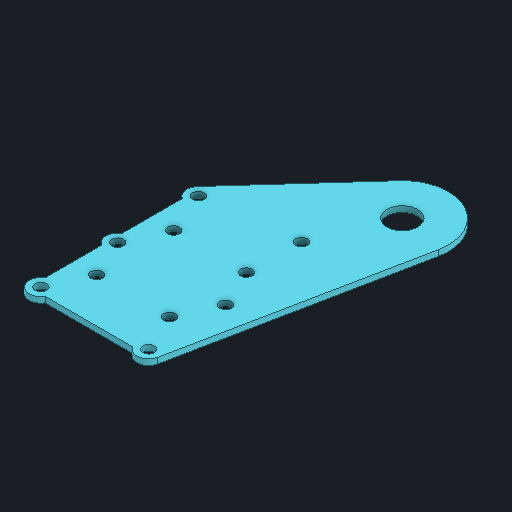
# Autodesk Inventor part: femur_support_steel
Saved by Autodesk Inventor 2026 (Build 300175000, 175)
## iProperties
Created: 2026-04-24
Part Number: femur_support_steel
Material: Сталь
Document SubType Name: Modeling
Designer: user
Density: 7.85 g/cm^3
Appearance: Серо-синий
Mass: 237.917 g
Surface Area: 222.677 cm^2
Volume: 30.3078 cm^3
Author: user
Autodesk Inventor part; units mm, degrees
ref_plane "YZ Plane" through (0, 0, 0) normal (1, 0, 0) x (0, 1, 0)
ref_plane "XZ Plane" through (0, 0, 0) normal (0, 1, 0) x (-1, 0, 0)
ref_plane "XY Plane" through (0, 0, 0) normal (0, 0, 1) x (1, 0, 0)
sketch "Эскиз1" plane through (0, 0, 0) normal (0, 1, 0) x (-1, 0, 0)
  circle A0 centre (41.8656, -145.8142) radius 8
  line L0 (111.6413, -105.8142) -> (38.7953, -105.8142) construction
  line L1 (76.8656, 21.9817) -> (76.8656, -112.0617)
  circle A1 centre (48.8156, -20.8142) radius 3.05
  circle A2 centre (57.9156, -40.8142) radius 3.05
  circle A3 centre (48.8156, -60.8142) radius 3.05
  circle A4 centre (57.9156, -80.8142) radius 3.05
  circle A5 centre (57.3656, -108.8642) radius 3.05
  circle A6 centre (104.9156, -102.7642) radius 3.05
  circle A7 centre (95.8156, -80.8142) radius 3.05
  circle A8 centre (104.9156, -60.8142) radius 3.05
  circle A9 centre (95.8156, -40.8142) radius 3.05
  circle A10 centre (104.9156, -20.8142) radius 3.05
  arc A11 (54.0984, -17.7642) -> (42.836, -19.6082) centre (48.8156, -20.8142) ccw
  arc A12 (107.9656, -26.0969) -> (99.6329, -17.7642) centre (104.9156, -20.8142) ccw
  arc A13 (107.9656, -66.0969) -> (107.9656, -55.5314) centre (104.9156, -60.8142) ccw
  arc A14 (109.4406, -106.855) -> (107.9656, -97.4814) centre (104.9156, -102.7642) ccw
  line L2 (107.9656, -97.4814) -> (107.9656, -66.0969)
  line L3 (107.9656, -55.5314) -> (107.9656, -26.0969)
  line L4 (99.6329, -17.7642) -> (54.0984, -17.7642)
  arc A15 (18.3393, -141.0693) -> (59.6688, -161.9091) centre (41.8656, -145.8142) ccw
  line L5 (59.6688, -161.9091) -> (109.4406, -106.855)
  line L6 (18.3393, -141.0693) -> (42.836, -19.6082)
  point P0 (0, 0)
  dimension "d4" = 37.9
  dimension "d5" = 56.1
  dimension "d6" = 6.1
  dimension "d7" = 45
  dimension "d8" = 40
  dimension "d9" = 25
  dimension "d10" = 40
  dimension "d11" = 37.9
  dimension "d12" = 56.1
  dimension "d15" = 35
  dimension "d16" = 40
  dimension "d17" = 16
  dimension "d18" = 19.5
  dimension "d20" = 12.2
  dimension "d21" = 12.2
  dimension "d22" = 12.2
  dimension "d23" = 3.05
  dimension "d24" = 3.05
  dimension "d25" = 48
  constraints: 16 centre point, 14 end point, 10 equal radius, 10 point on circle, 6 tangent, 5 coincident, 5 vertical alignment, 4 horizontal alignment, 2 point on line, 2 vertical, 1 horizontal, 1 perpendicular, 1 other
  measures "d4" distance of A7.centre A4.centre
  measures "d5" distance of A10.centre A1.centre
  measures "d6" diameter of A1
  measures "d7" distance from line of A3.centre L0
  measures "d8" distance of A1.centre A3.centre
  measures "d9" distance from line of L0 A4.centre
  measures "d10" distance of A2.centre A4.centre
  measures "d11" diameter of A2.centre L1
  measures "d12" diameter of A1.centre L1
  measures "d15" distance from line of A0.centre L1
  measures "d16" distance from line of L0 A0.centre
  measures "d17" diameter of A0
  measures "d18" distance from line of A5.centre L1
  measures "d20" diameter of A12
  measures "d21" diameter of A13
  measures "d22" diameter of A14
  measures "d23" distance from line of L2 A6.centre
  measures "d24" distance from line of L4 A10.centre
  measures "d25" diameter of A15
extrude "Выдавливание1" add sketch "Эскиз1" along normal blind 3
equation "\"d4\" = -d_main_screw_holes + hight_profile_femur - 2 * thickness_profile_femur"
equation "\"d5\" = hight_profile_femur + d_main_screw_holes"
equation "\"d6\" = d_main_screw_holes"
equation "\"d11\" = -d_main_screw_holes + hight_profile_femur - 2 * thickness_profile_femur"
equation "\"d12\" = hight_profile_femur + d_main_screw_holes"
equation "\"d15\" = width_shaft_shift"
equation "\"d16\" = hight_shaft_shift"
equation "\"d17\" = d_main_shaft"
equation "\"d20\" = 2 * d_main_screw_holes"
equation "\"d21\" = 2 * d_main_screw_holes"
equation "\"d22\" = 2 * d_main_screw_holes"
equation "\"d23\" = 0.5 * d_main_screw_holes"
equation "\"d24\" = 0.5 * d_main_screw_holes"
equation "\"d2\" = thickness_steel"
equation "\"tolerance_plazma\" = 0.1"
equation "\"thickness_steel\" = 3"
equation "\"d_main_screw_holes\" = 6.1"
equation "\"d_main_shaft\" = 16"
equation "\"thickness_profile_tibea\" = 4"
equation "\"hight_shaft_shift\" = 40"
equation "\"thickness_profile_femur\" = 3"
equation "\"width_shaft_shift\" = 35"
equation "\"hight_profile_femur\" = 50"
equation "\"width_flattened_surface\" = 12"
